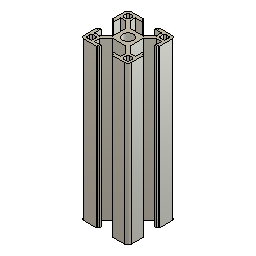
30X30 - T-slot - Aluminium Profile (Autodesk Fusion 360 design; units mm, degrees)
Autodesk Fusion 360 part; units mm, degrees
sketch "Sketch1" plane through (0, 0, 0) normal (0, 1, 0) x (1, 0, 0)
  circle A0 centre (0, 0) radius 3.4
  line L0 (5.8, -4.25) -> (5.8, 4.25)
  line L1 (4.4302, 5.8) -> (-4.0698, 5.8)
  line L2 (-5.8, 4.25) -> (-5.8, -4.25)
  arc A1 (-13, 15) -> (-15, 13) centre (-13, 13) ccw
  arc A2 (15, 13) -> (13, 15) centre (13, 13) ccw
  arc A3 (12.9984, -15) -> (15, -13) centre (13, -13) ccw
  arc A4 (-15, -13.001) -> (-13, -15) centre (-13, -13) ccw
  line L3 (-9.0785, 8.25) -> (-13, 8.25)
  line L4 (-10.4448, -8.25) -> (-13, -8.25)
  line L5 (-8.25, 10.6606) -> (-8.25, 13)
  line L6 (8.25, 9.241) -> (8.25, 13)
  line L7 (-12.5, 9.75) -> (-10.75, 9.75)
  line L8 (-9.75, 10.75) -> (-9.75, 12.5)
  line L9 (-10.75, 13.5) -> (-12.5, 13.5)
  line L10 (-13.5, 12.5) -> (-13.5, 10.75)
  arc A5 (-12.5, 13.5) -> (-13.5, 12.5) centre (-12.5, 12.5) ccw
  arc A6 (-9.75, 12.5) -> (-10.75, 13.5) centre (-10.75, 12.5) ccw
  arc A7 (-10.75, 9.75) -> (-9.75, 10.75) centre (-10.75, 10.75) ccw
  arc A8 (-13.5, 10.75) -> (-12.5, 9.75) centre (-12.5, 10.75) ccw
  line L11 (-4.1, 14) -> (-5.1, 14)
  line L12 (-5.1, 14) -> (-5.1, 15)
  line L13 (4.1, 13) -> (4.1, 14)
  line L14 (4.1, 14) -> (5.1, 14)
  line L15 (5.1, 14) -> (5.1, 15)
  line L16 (-4.1, 14) -> (-4.1, 13)
  line L17 (0, 15) -> (0, -15) construction
  line L18 (-15, 0) -> (15, 0) construction
  line L19 (13.5, 12.5) -> (13.5, 10.75)
  line L20 (12.5, 9.75) -> (10.75, 9.75)
  arc A9 (10.75, 13.5) -> (9.75, 12.5) centre (10.75, 12.5) ccw
  arc A10 (9.75, 10.75) -> (10.75, 9.75) centre (10.75, 10.75) ccw
  line L21 (9.75, 10.75) -> (9.75, 12.5)
  arc A11 (12.5, 9.75) -> (13.5, 10.75) centre (12.5, 10.75) ccw
  line L22 (10.75, 13.5) -> (12.5, 13.5)
  arc A12 (13.5, 12.5) -> (12.5, 13.5) centre (12.5, 12.5) ccw
  arc A13 (-9.75, -10.75) -> (-10.75, -9.75) centre (-10.75, -10.75) ccw
  line L23 (-9.75, -10.75) -> (-9.75, -12.5)
  line L24 (-13.5, -12.5) -> (-13.5, -10.75)
  line L25 (-10.75, -13.5) -> (-12.5, -13.5)
  arc A14 (-13.5, -12.5) -> (-12.5, -13.5) centre (-12.5, -12.5) ccw
  line L26 (-12.5, -9.75) -> (-10.75, -9.75)
  arc A15 (-12.5, -9.75) -> (-13.5, -10.75) centre (-12.5, -10.75) ccw
  arc A16 (-10.75, -13.5) -> (-9.75, -12.5) centre (-10.75, -12.5) ccw
  arc A17 (12.5, -13.5) -> (13.5, -12.5) centre (12.5, -12.5) ccw
  arc A18 (10.75, -9.75) -> (9.75, -10.75) centre (10.75, -10.75) ccw
  arc A19 (9.75, -12.5) -> (10.75, -13.5) centre (10.75, -12.5) ccw
  line L27 (9.75, -10.75) -> (9.75, -12.5)
  line L28 (12.5, -9.75) -> (10.75, -9.75)
  arc A20 (13.5, -10.75) -> (12.5, -9.75) centre (12.5, -10.75) ccw
  line L29 (13.5, -12.5) -> (13.5, -10.75)
  line L30 (10.75, -13.5) -> (12.5, -13.5)
  line L31 (-4.1, -14) -> (-5.1, -14)
  line L32 (-4.1, -14) -> (-4.1, -13)
  line L33 (-5.1, -14) -> (-5.1, -15)
  line L34 (4.1, -13) -> (4.1, -14)
  line L35 (4.1, -14) -> (5.1, -14)
  line L36 (5.1, -14) -> (5.1, -15)
  line L37 (-8.25, -10.6606) -> (-8.25, -13)
  line L38 (-13, -15) -> (-5.1, -15)
  line L39 (5.1, -15) -> (12.9984, -15)
  line L40 (-8.25, -13) -> (-4.1, -13)
  line L41 (13, 15) -> (5.1, 15)
  line L42 (-5.1, 15) -> (-13, 15)
  line L43 (8.25, 13) -> (4.1, 13)
  line L44 (-4.1, 13) -> (-8.25, 13)
  line L45 (8.25, -9.768) -> (8.25, -13)
  line L46 (-13, -13) -> (12.5, 12.5) construction
  line L47 (-12.5, 12.5) -> (13, -13) construction
  line L48 (13, -8.25) -> (9.8438, -8.25)
  line L49 (5.8, -4.25) -> (9.8438, -8.25)
  line L50 (4.1, -13) -> (8.25, -13)
  line L51 (13, 8.25) -> (9.3051, 8.25)
  line L52 (-4.2601, -5.7908) -> (4.2399, -5.7908)
  line L53 (-13, 4.1) -> (-14, 4.1)
  line L54 (-14, 4.1) -> (-14, 5.1)
  line L55 (-14, 5.1) -> (-15, 5.1)
  line L56 (-13, -4.1) -> (-14, -4.1)
  line L57 (-14, -4.1) -> (-14, -5.1)
  line L58 (-14, -5.1) -> (-15, -5.1)
  line L59 (-13, 8.25) -> (-13, 4.1)
  line L60 (-13, -4.1) -> (-13, -8.25)
  line L61 (-15, 13) -> (-15, 5.1)
  line L62 (-15, -5.1) -> (-15, -13.001)
  line L63 (13, -8.25) -> (13, -3.9838)
  line L64 (13, 4.0895) -> (13, 10.5589)
  line L65 (15, -13) -> (15, -4.9838)
  line L66 (15, 5.0895) -> (15, 13)
  dimension "d1" = 6.8
  dimension "d2" = 30
  dimension "d3" = 30
  dimension "d5" = 9.2
  dimension "d6" = 9.2
  dimension "d7" = 9.2
  dimension "d13" = 2
  dimension "d14" = 2
  dimension "d15" = 2
  dimension "d16" = 2
  dimension "d17" = 16.5
  dimension "d19" = 16.5
  dimension "d22" = 1.5
  dimension "d23" = 1.5
  dimension "d24" = 1.5
  dimension "d25" = 1.5
  dimension "d26" = 1
  dimension "d33" = 4.1
  dimension "d34" = 1
  dimension "d35" = 2
  dimension "d36" = 2
  dimension "d37" = 2
  dimension "d39" = 3.75
  dimension "d40" = 3.75
  dimension "d41" = 5.8
  dimension "d42" = 5.8
  dimension "d43" = 5.8
  dimension "d45" = 8.5
  dimension "d46" = 8.5
  dimension "d48" = 8.5
  dimension "d49" = 1
  dimension "d51" = 8.2
  dimension "d52" = 1.5
  dimension "d53" = 1.5
  dimension "d54" = 1.5
  dimension "d55" = 1.5
  dimension "d57" = 1.5
  dimension "d58" = 1.5
  dimension "d59" = 4.25
  dimension "d60" = 4.25
  dimension "d64" = 8.5
  dimension "d65" = 1
  dimension "d66" = 1
  dimension "d67" = 1
  dimension "d68" = 1
  dimension "d71" = 8.2
  dimension "d72" = 4.1
  measures "d1" diameter of A0
  measures "d5" distance of L0 L65
  measures "d6" distance of L2 L61
  measures "d7" distance of L1 L41
  measures "d13" radius of A1
  measures "d14" radius of A2
  measures "d15" radius of A3
  measures "d16" radius of A4
  measures "d17" distance of L3 L4
  measures "d19" distance of L5 L6
  measures "d22" distance of L5 L8
  measures "d23" distance of L10 L61
  measures "d24" distance of L3 L7
  measures "d25" distance of L9 L41
  measures "d26" radius of A5
  measures "d33" distance of L13
  measures "d35" distance of L41 L43
  measures "d36" distance of L59 L61
  measures "d37" distance of L63 L65
  measures "d39" distance of L8 L10
  measures "d40" distance of L7 L9
  measures "d41" distance of L1
  measures "d42" distance of L2
  measures "d43" distance of L0
  measures "d51" distance of L13 L16
  measures "d52" distance of L23 L37
  measures "d53" distance of L4 L26
  measures "d54" distance of L27 L45
  measures "d55" distance of L28 L48
  measures "d57" distance of L20 L51
  measures "d58" distance of L6 L21
  measures "d59" distance of L18
  measures "d60" distance of L18
  measures "d71" distance of L53 L56
  measures "d72" distance of L18 L53
sketch "Sketch2" plane through (0, 0, 0) normal (0, 1, 0) x (-1, 0, 0)
  line L0 (13, -8.25) -> (13, -4.1)
  line L1 (13, -4.1) -> (14, -4.1)
  line L2 (13, -4.1) -> (14, -4.1)
  line L3 (14, -4.1) -> (14, -5.1)
  line L4 (14, -5.1) -> (15, -5.1)
  line L5 (15, -5.1) -> (15, -13)
  line L6 (5.1, -15) -> (13, -15)
  line L7 (13, -15) -> (5.1, -15)
  line L8 (5.1, -14) -> (4.1, -14)
  line L9 (4.1, -14) -> (4.1, -13)
  line L10 (4.1, -13) -> (8.25, -13)
  arc A0 (13, -15) -> (15, -13) centre (13, -13) ccw
  line L11 (12.5, -13.5) -> (10.75, -13.5)
  line L12 (9.75, -12.5) -> (9.75, -10.75)
  line L13 (10.75, -9.75) -> (12.5, -9.75)
  line L14 (13.5, -10.75) -> (13.5, -12.5)
  arc A1 (12.5, -13.5) -> (13.5, -12.5) centre (12.5, -12.5) ccw
  line L15 (12.5, -12.5) -> (-13, 13)
  arc A2 (12.5, -13.5) -> (13.5, -12.5) centre (12.5, -12.5) ccw
  arc A3 (9.75, -12.5) -> (10.75, -13.5) centre (10.75, -12.5) ccw
  arc A4 (10.75, -9.75) -> (9.75, -10.75) centre (10.75, -10.75) ccw
  arc A5 (13.5, -10.75) -> (12.5, -9.75) centre (12.5, -10.75) ccw
  line L16 (15, -13) -> (15, -5.1)
  line L17 (12.5, -9.75) -> (10.75, -9.75)
  line L18 (10.75, -13.5) -> (12.5, -13.5)
  line L19 (9.5009, -9.5009) -> (1.6153, -1.6153) construction
  line L20 (8.25, -13) -> (8.25, -9.6642)
  line L21 (8.25, -10.6606) -> (8.25, -13)
  line L22 (13, -8.25) -> (9.6642, -8.25)
  line L23 (5.1, -14) -> (5.1, -15)
  line L24 (9.6642, -8.25) -> (5.5142, -4.1)
  line L25 (8.25, -9.6642) -> (4.1, -5.5142)
  line L26 (13.5, 10.75) -> (13.5, 12.5)
  arc A6 (13.5, 12.5) -> (12.5, 13.5) centre (12.5, 12.5) ccw
  arc A7 (10.75, 13.5) -> (9.75, 12.5) centre (10.75, 12.5) ccw
  line L27 (9.75, 12.5) -> (9.75, 10.75)
  line L28 (9.5009, 9.5009) -> (1.6153, 1.6153) construction
  line L29 (13, 8.25) -> (13, 4.1)
  arc A8 (9.75, 10.75) -> (10.75, 9.75) centre (10.75, 10.75) ccw
  line L30 (13, 4.1) -> (14, 4.1)
  arc A9 (13.5, 12.5) -> (12.5, 13.5) centre (12.5, 12.5) ccw
  line L31 (13, 4.1) -> (14, 4.1)
  line L32 (14, 4.1) -> (14, 5.1)
  line L33 (14, 5.1) -> (15, 5.1)
  line L34 (10.75, 9.75) -> (12.5, 9.75)
  line L35 (12.5, 9.75) -> (10.75, 9.75)
  line L36 (13, 8.25) -> (9.6642, 8.25)
  arc A10 (12.5, 9.75) -> (13.5, 10.75) centre (12.5, 10.75) ccw
  line L37 (4.1, 14) -> (4.1, 13)
  line L38 (5.1, 14) -> (4.1, 14)
  line L39 (15, 13) -> (15, 5.1)
  line L40 (15, 5.1) -> (15, 13)
  line L41 (5.1, 15) -> (13, 15)
  line L42 (13, 15) -> (5.1, 15)
  line L43 (4.1, 13) -> (8.25, 13)
  line L44 (12.5, 13.5) -> (10.75, 13.5)
  line L45 (10.75, 13.5) -> (12.5, 13.5)
  line L46 (8.25, 13) -> (8.25, 9.6642)
  line L47 (9.6642, 8.25) -> (5.5142, 4.1)
  line L48 (8.25, 10.6606) -> (8.25, 13)
  arc A11 (15, 13) -> (13, 15) centre (13, 13) ccw
  line L49 (8.25, 9.6642) -> (4.1, 5.5142)
  line L50 (5.1, 14) -> (5.1, 15)
  line L51 (-8.25, 9.6642) -> (-4.1, 5.5142)
  line L52 (-8.25, 10.6606) -> (-8.25, 13)
  line L53 (-12.5, -13.5) -> (-10.75, -13.5)
  arc A12 (-10.75, 9.75) -> (-9.75, 10.75) centre (-10.75, 10.75) ccw
  line L54 (-8.25, 13) -> (-8.25, 9.6642)
  line L55 (-4.1, -13) -> (-8.25, -13)
  line L56 (-15, -5.1) -> (-15, -13)
  line L57 (-9.75, 12.5) -> (-9.75, 10.75)
  line L58 (-13, -8.25) -> (-13, -4.1)
  line L59 (-8.25, -10.6606) -> (-8.25, -13)
  line L60 (-13, 8.25) -> (-13, 4.1)
  line L61 (-12.5, 13.5) -> (-10.75, 13.5)
  line L62 (-4.1, 13) -> (-8.25, 13)
  line L63 (-4.1, -14) -> (-4.1, -13)
  line L64 (-13, -15) -> (-5.1, -15)
  line L65 (-13.5, 10.75) -> (-13.5, 12.5)
  line L66 (-8.25, -13) -> (-8.25, -9.6642)
  line L67 (-9.6642, 8.25) -> (-5.5142, 4.1)
  arc A13 (-12.5, 13.5) -> (-13.5, 12.5) centre (-12.5, 12.5) ccw
  line L68 (-10.75, 13.5) -> (-12.5, 13.5)
  arc A14 (-13.5, -12.5) -> (-12.5, -13.5) centre (-12.5, -12.5) ccw
  line L69 (-13, -8.25) -> (-9.6642, -8.25)
  arc A15 (-12.5, -9.75) -> (-13.5, -10.75) centre (-12.5, -10.75) ccw
  arc A16 (-10.75, -13.5) -> (-9.75, -12.5) centre (-10.75, -12.5) ccw
  line L70 (-14, 5.1) -> (-15, 5.1)
  line L71 (-14, -5.1) -> (-15, -5.1)
  line L72 (-13, 15) -> (-5.1, 15)
  line L73 (-10.75, 9.75) -> (-12.5, 9.75)
  line L74 (-13, -4.1) -> (-14, -4.1)
  line L75 (-5.1, -14) -> (-5.1, -15)
  line L76 (-14, 4.1) -> (-14, 5.1)
  arc A17 (-9.75, -10.75) -> (-10.75, -9.75) centre (-10.75, -10.75) ccw
  line L77 (-14, -4.1) -> (-14, -5.1)
  line L78 (-15, 13) -> (-15, 5.1)
  line L79 (-10.75, -13.5) -> (-12.5, -13.5)
  line L80 (-13.5, -10.75) -> (-13.5, -12.5)
  line L81 (-5.1, -15) -> (-13, -15)
  arc A18 (-9.75, 12.5) -> (-10.75, 13.5) centre (-10.75, 12.5) ccw
  line L82 (-13, 4.1) -> (-14, 4.1)
  line L83 (-13, -4.1) -> (-14, -4.1)
  line L84 (-5.1, 14) -> (-5.1, 15)
  line L85 (-8.25, -9.6642) -> (-4.1, -5.5142)
  line L86 (-13, 4.1) -> (-14, 4.1)
  arc A19 (-13.5, 10.75) -> (-12.5, 9.75) centre (-12.5, 10.75) ccw
  line L87 (-15, -13) -> (-15, -5.1)
  line L88 (-9.5009, 9.5009) -> (-1.6152, 1.6153) construction
  line L89 (-10.75, -9.75) -> (-12.5, -9.75)
  line L90 (-5.1, 14) -> (-4.1, 14)
  line L91 (-15, 5.1) -> (-15, 13)
  line L92 (-9.75, -12.5) -> (-9.75, -10.75)
  arc A20 (-13, 15) -> (-15, 13) centre (-13, 13) ccw
  line L93 (-12.5, -9.75) -> (-10.75, -9.75)
  arc A21 (-15, -13) -> (-13, -15) centre (-13, -13) ccw
  arc A22 (-13.5, -12.5) -> (-12.5, -13.5) centre (-12.5, -12.5) ccw
  arc A23 (-12.5, 13.5) -> (-13.5, 12.5) centre (-12.5, 12.5) ccw
  line L94 (-5.1, -14) -> (-4.1, -14)
  line L95 (-12.5, 9.75) -> (-10.75, 9.75)
  line L96 (-9.5009, -9.5009) -> (-1.6152, -1.6153) construction
  line L97 (-5.1, 15) -> (-13, 15)
  line L98 (-13, 8.25) -> (-9.6642, 8.25)
  line L99 (-9.6642, -8.25) -> (-5.5142, -4.1)
  line L100 (-4.1, 14) -> (-4.1, 13)
  line L101 (4.1, -5.5142) -> (-4.1, -5.5142)
  line L102 (5.5142, 4.1) -> (5.5142, -4.1)
  line L103 (-5.5142, 4.1) -> (-5.5142, -4.1)
  line L104 (4.1, 5.5142) -> (-4.1, 5.5142)
  circle A24 centre (0, 0) radius 3.4
  dimension "d78" = 2
  dimension "d79" = 1
  dimension "d80" = 1.5
  dimension "d91" = 1
  dimension "d92" = 1
  dimension "d93" = 1.5
  dimension "d94" = 1.5
  dimension "d102" = 3.75
  dimension "d103" = 1.5
  dimension "d104" = 3.75
  dimension "d105" = 2
  dimension "d106" = 2
  dimension "d109" = 5.869
  dimension "d110" = 5.869
  dimension "d111" = 3.3358
  dimension "d112" = 3.3358
  dimension "d113" = 4.15
  dimension "d114" = 4.15
  dimension "d115" = 8.2
  dimension "d116" = 8.2
  dimension "d117" = 8.2
  dimension "d118" = 8.2
  dimension "d119" = 6.8
  measures "d78" radius of A0
  measures "d79" radius of A2
  measures "d80" distance of L14 L16
  measures "d91" distance of L19 L24
  measures "d92" distance of L15 L25
  measures "d93" distance of L12 L20
  measures "d94" distance of L13 L22
  measures "d102" distance of L12 L14
  measures "d103" distance of L7 L11
  measures "d104" distance of L11 L13
  measures "d105" distance of L7 L10
  measures "d106" distance of L0 L5
  measures "d119" diameter of A24
extrude "Extrude1" add sketch "Sketch2" along normal blind 100
equation "d33 = ( 8.2 / 2 ) * 1 mm"
equation "d59 = ( 8.5 / 2 ) * 1 mm"
equation "d60 = ( 8.5 / 2 ) * 1 mm"
equation "d72 = ( 8.2 / 2 ) * 1 mm"
equation "Length = 100.00 mm"
